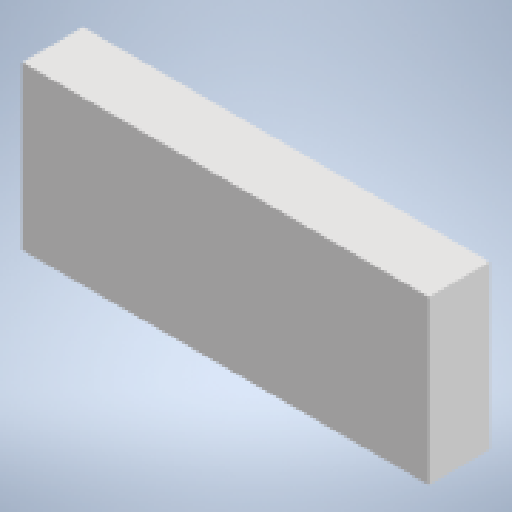
# Autodesk Inventor part: chwyt
Saved by Autodesk Inventor 2025.2 (Build 292293000, 293)
## iProperties
Created: 2026-05-08
Part Number: chwyt
Material: Ogólny
Document SubType Name: Modeling
Designer: muszy
Density: 1 g/cm^3
Appearance: Domyślna
Author: muszy
Autodesk Inventor part; units mm, degrees
ref_plane "YZ Plane" through (0, 0, 0) normal (1, 0, 0) x (0, 1, 0)
ref_plane "XZ Plane" through (0, 0, 0) normal (0, 1, 0) x (-1, 0, 0)
ref_plane "XY Plane" through (0, 0, 0) normal (0, 0, 1) x (1, 0, 0)
sketch "Szkic1" plane through (0, 0, 0) normal (0, 0, 1) x (1, 0, 0)
  line L0 (-10, 4) -> (10, 4)
  line L1 (10, 4) -> (10, -4)
  line L2 (10, -4) -> (-10, -4)
  line L3 (-10, -4) -> (-10, 4)
  line L4 (-10, 4) -> (10, -4) construction
  line L5 (10, 4) -> (-10, -4) construction
  point P0 (0, 0)
  dimension "d0" = 8
  dimension "d1" = 20
  constraints: 12 end point, 2 midpoint, 2 parallel, 1 horizontal, 1 perpendicular
  measures "d0" distance between parallel lines of L2 L0
  measures "d1" distance between parallel lines of L3 L1
extrude "Wyciągnięcie proste1" add sketch "Szkic1" along normal blind 3
sketch "Szkic2" plane through (0, 0, 3) normal (0, 0, 1) x (1, 0, 0)
  line L0 (-10, 4) -> (-10, -4) projected
  point P0 (0, 0)
  point P1 (-4, 0)
  point P2 (4, 0)
  dimension "d6" = 8
  dimension "d7" = 6
  measures "d6" distance of point (4, 0) point (-4, 0)
  measures "d7" distance from line of L0 point (-4, 0)
hole "Otwór1" at (-4, 0, 3) at (4, 0, 3) direction (0, 0, -1) diameter 4.134 depth 7 tip angle 118 countersink diameter 7 countersink angle 90 thread size "M5x0.8" class "6H" standard "ISO Metric profile"
sketch "Szkic3" plane through (0, 0, 3) normal (0, 0, 1) x (1, 0, 0)
  line L0 (10, 4) -> (-10, 4) projected
  line L1 (-10, -4) -> (10, -4) projected
  line L2 (10, 4) -> (7.6326, 4)
  line L3 (7.6326, 4) -> (7.6326, -4)
  line L4 (7.6326, -4) -> (10, -4)
  line L5 (10, -4) -> (10, 4)
  point P0 (0, 0)
  point P1 (10, -4)
  constraints: 8 end point, 2 parallel, 1 horizontal, 1 perpendicular, 1 point on line
extrude "Wyciągnięcie proste2" add sketch "Szkic3" along normal blind 1
sketch "Szkic4" plane through (0, 0, 4) normal (0, 0, 1) x (1, 0, 0)
  line L0 (10, -4) -> (10, 4) projected
  line L1 (10, -4) -> (7.633, -4)
  line L2 (7.633, -4) -> (7.633, 26)
  line L3 (7.633, 26) -> (10, 26)
  line L4 (10, 26) -> (10, -4)
  point P0 (0, 0)
  dimension "d17" = 2.367
  dimension "d18" = 30
  constraints: 8 end point, 2 parallel, 1 horizontal, 1 perpendicular
  measures "d17" distance between parallel lines of L2 L0
  measures "d18" distance between parallel lines of L1 L3
extrude "Wyciągnięcie proste3" add sketch "Szkic4" along normal blind 20
